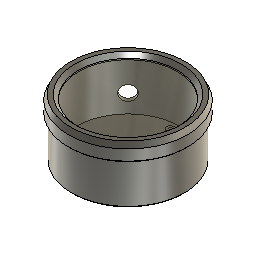
Gauge (Autodesk Fusion 360 design; units mm, degrees)
Autodesk Fusion 360 part; units mm, degrees
sketch "Sketch1" plane through (0, 0, 0) normal (0, 0, 1) x (1, 0, 0)
  circle A0 centre (0, 0) radius 42.5
  circle A1 centre (0, 0) radius 46.5
  dimension "d1" = 85
  dimension "d2" = 93
  constraint coincident A0.centre A1.centre
  constraint concentric A0 A1
  measures "d1" diameter of A0
  measures "d2" diameter of A1
extrude "Extrude1" add sketch "Sketch1" along normal blind 40 makes body 1
extrude "Extrude2" add sketch "Sketch1" against normal blind 4 contours A0 | A1 bodies 1
ref_plane "WorkPlane1" through (0, 0, 40) normal (0, 0, 1) x (1, 0, 0)
sketch "Sketch3" plane through (0, 0, 40) normal (0, 0, 1) x (1, 0, 0)
  circle A0 centre (0, 0) radius 46.5
  circle A1 centre (0, 0) radius 42.5
  circle A2 centre (0, 0) radius 49
  circle A3 centre (0, 0) radius 40.5
  circle A4 centre (0, 0) radius 46.7
  circle A5 centre (0, 0) radius 46.3
  dimension "d9" = 98
  dimension "d10" = 81
  dimension "d50" = 0.2
  dimension "d53" = -0.2
  constraint concentric A0 A2
  constraint concentric A0 A3
  measures "d9" diameter of A2
  measures "d10" diameter of A3
extrude "Extrude3" add sketch "Sketch3" along normal blind 4 separate body contours A0 | A1 | A2 | A4 | A5 makes body 2
extrude "Extrude4" add sketch "Sketch3" against normal blind 10 contours A2 bodies 2
chamfer "Chamfer1" distance 3 angle 45 1 edges at (-37.7593, 14.6454, 44) on bodies 2
chamfer "Chamfer2" distance 2 angle 65 1 edges at (-45.684, -17.7192, 44) measured on face at (46.8223, -4.5955, 44) on bodies 2
chamfer "Chamfer3" distance 1 angle 45 1 edges at (-45.684, 17.7192, 30) measured on face at (47.877, -4.7544, 30) on bodies 2
chamfer "Chamfer4" distance 1 angle 45 1 edges at (-43.3532, 16.8151, -4) measured on face at (10.204, -8.5364, -4) on bodies 1
ref_plane "WorkPlane2" through (0, 0, 6) normal (0, 0, 1) x (1, 0, 0)
sketch "Sketch4" plane through (0, 0, 6) normal (0, 0, 1) x (1, 0, 0)
  line L0 (0, 0) -> (67.9412, 0) construction
  circle A0 centre (0, 0) radius 46.5 construction
  line L1 (-25.8948, 38.6227) -> (-38.6227, 25.8948)
  line L2 (-38.6227, 25.8948) -> (-54.1711, 36.1937)
  line L3 (-54.1711, 36.1937) -> (-37.6611, 54.4375)
  line L4 (-37.6611, 54.4375) -> (-25.8948, 38.6227)
  line L5 (0, 0) -> (-64.5174, 64.5174) construction
  line L6 (0, 0) -> (62.2977, 0) construction
  dimension "d26" = 18
  dimension "d27" = 135
  constraint horizontal L0
  constraint coincident L0.start A0.centre
  constraint coincident A0 L1.start
  constraint coincident A0 L1.end
  constraint horizontal L6
  constraint midpoint L1 L5
  measures "d26" distance of L1.start L1.end
  measures "d27" angle of L5 L6
extrude "Extrude5" cut sketch "Sketch4" along normal blind 18 bodies 1 2
sketch "Sketch5" plane through (-32.2587, 32.2587, 0) normal (-0.707107, 0.707107, 0) x (-0.707107, -0.707107, 0)
  line L0 (-9, 6) -> (9, 6)
  line L1 (9, 6) -> (9, 24)
  line L2 (9, 24) -> (-9, 24)
  line L3 (-9, 24) -> (-9, 6)
  circle A0 centre (0, 15) radius 6
  dimension "d30" = 12
  measures "d30" diameter of A0
extrude "Extrude6" cut sketch "Sketch5" against normal blind 15 contours A0 bodies 1
sketch "Sketch6" plane through (0, 0, 0) normal (0, 0, 1) x (-1, 0, 0)
  circle A0 centre (0, 0) radius 42.5
  circle A1 centre (0, -35) radius 3
  circle A2 centre (30.31, 17.5) radius 3
  circle A3 centre (-30.31, 17.5) radius 3
  circle A4 centre (0, 0) radius 4
  dimension "d33" = 6
  dimension "d34" = 6
  dimension "d35" = 6
  dimension "d36" = 35
  dimension "d37" = 17.5
  dimension "d38" = 17.5
  dimension "d39" = 30.31
  dimension "d40" = 30.31
  dimension "d42" = 8
  constraint vertical A0.centre A1.centre
  constraint coincident A0.centre A4.centre
  measures "d33" diameter of A2
  measures "d34" diameter of A3
  measures "d35" diameter of A1
  measures "d36" distance of A0.centre A1.centre
  measures "d37" vertical distance of A0.centre A2.centre
  measures "d38" vertical distance of A0.centre A3.centre
  measures "d39" horizontal distance of A0.centre A3.centre
  measures "d40" horizontal distance of A0.centre A2.centre
  measures "d42" diameter of A4
extrude "Extrude7" cut sketch "Sketch6" against normal through all contours A4 bodies 1
extrude "Extrude8" add sketch "Sketch6" along normal blind 2 contours A1 | A2 | A3 bodies 1
sketch "Sketch7" plane through (0, 0, 2) normal (0, 0, 1) x (-1, 0, 0)
  circle A0 centre (0, -35) radius 3
  circle A1 centre (0, -35) radius 1
  circle A2 centre (30.31, 17.5) radius 1
  circle A3 centre (-30.31, 17.5) radius 1
  point P0 (30.31, 17.5)
  point P1 (-30.31, 17.5)
  dimension "d45" = 2
  dimension "d46" = 2
  dimension "d47" = 2
  constraint concentric A0 A1
  constraint coincident P0 A2.centre
  constraint coincident P1 A3.centre
  measures "d45" diameter of A1
  measures "d46" diameter of A2
  measures "d47" diameter of A3
extrude "Extrude9" cut sketch "Sketch7" against normal through all contours A1 | A2 | A3 bodies 1
chamfer "Chamfer5" distance 1 angle 45 1 edges at (-43.3532, -16.8151, 40) measured on face at (44.8353, -4.4216, 40) on bodies 1
extrude "Extrude10" add sketch "Sketch3" along normal blind 1 separate body contours A1 | A3 | A5 makes body 3
